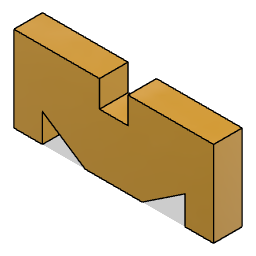
3d08 v1 (Autodesk Fusion 360 design; units mm, degrees)
Autodesk Fusion 360 part; units mm, degrees
sketch "Sketch1" plane through (0, 0, 0) normal (0, 0, 1) x (1, 0, 0)
  line L0 (0, 0) -> (0, 30)
  line L1 (0, 30) -> (30, 30)
  line L2 (30, 30) -> (30, 20.7071)
  line L3 (30, 20.7071) -> (40, 20.7071)
  line L4 (40, 20.7071) -> (40, 30)
  line L5 (40, 30) -> (70, 30)
  line L6 (70, 30) -> (70, 0)
  line L7 (60, 0) -> (60, 10)
  line L8 (60, 10) -> (45, 0)
  line L9 (45, 0) -> (25, 0)
  line L10 (25, 0) -> (10, 10)
  line L11 (10, 10) -> (10, 0)
  line L12 (10, 0) -> (0, 0)
  line L13 (60, 0) -> (70, 0)
  dimension "d1" = 30
  dimension "d4" = 30
  dimension "d5" = 30
  dimension "d9" = 70
  dimension "d10" = 10
  dimension "d11" = 15
  dimension "d12" = 20
  dimension "d13" = 10
  dimension "d14" = 15
  dimension "d15" = 10
  dimension "d16" = 30
  dimension "d17" = 10
  dimension "d18" = 10
  dimension "d19" = 20.7071
  dimension "d20" = 90
  dimension "d21" = 112.62
  constraint coincident L0.start L12.end
  constraint vertical L0
  constraint perpendicular L0 L1
  constraint perpendicular L1 L2
  constraint perpendicular L2 L3
  constraint perpendicular L3 L4
  constraint perpendicular L4 L5
  constraint perpendicular L5 L6
  constraint perpendicular L5 L7
  constraint perpendicular L6 L9
  constraint perpendicular L0 L12
  constraint horizontal L0.start L6.end
  constraint perpendicular L6 L13
  measures "d1" distance of L0.end L1.end
  measures "d4" distance of L0.start L0.end
  measures "d5" distance of L5.end L6.end
  measures "d9" distance of L0.start L6.end
  measures "d10" distance of L11.end L0.start
  measures "d11" distance of L9.end L11.end
  measures "d12" distance of L8.end L9.end
  measures "d13" distance of L6.end L7.start
  measures "d14" distance of L7.start L8.end
  measures "d15" distance of L2.end L3.end
  measures "d16" distance of L4.end L5.end
  measures "d17" distance of L10.end L11.end
  measures "d18" distance of L7.start L7.end
  measures "d19" distance of L0.start L3
  measures "d20" angle of L9 L11
  measures "d21" angle of L8 L10
extrude "Extrude1" add sketch "Sketch1" along normal mid plane 10
